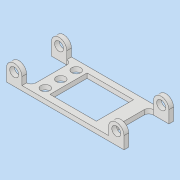
# Autodesk Inventor part: RelayHolder
Saved by Autodesk Inventor 2017 (Build 210142000, 142)
## iProperties
Created: 2018-03-03
Part Number: RelayHolder
Material: ABS Plastic
Document SubType Name: Modeling
Designer: Derek Wider
Density: 1.06 g/cm^3
Appearance: Smooth - White
Author: Derek Wider
Autodesk Inventor part; units mm, degrees
ref_plane "YZ Plane" through (0, 0, 0) normal (1, 0, 0) x (0, 1, 0)
ref_plane "XZ Plane" through (0, 0, 0) normal (0, 1, 0) x (-1, 0, 0)
ref_plane "XY Plane" through (0, 0, 0) normal (0, 0, 1) x (1, 0, 0)
sketch "Sketch1" plane through (0, 0, 0) normal (0, 1, 0) x (-1, 0, 0)
  line L0 (0, 0) -> (48.26, 0)
  line L1 (48.26, 0) -> (48.26, -20.32)
  line L2 (48.26, -20.32) -> (0, -20.32)
  line L3 (0, -20.32) -> (0, 0)
  line L4 (33.02, -2.6035) -> (13.97, -2.6035)
  line L5 (13.97, -2.6035) -> (13.97, -17.8435)
  line L6 (13.97, -17.8435) -> (33.02, -17.8435)
  line L7 (33.02, -17.8435) -> (33.02, -2.6035)
  dimension "d0" = 48.26
  dimension "d1" = 20.32
  dimension "d2" = 19.05
  dimension "d3" = 15.24
  dimension "d4" = 15.24
  dimension "d5" = 2.6035
  constraints: 16 end point, 4 parallel, 2 horizontal, 2 perpendicular
  measures "d0" distance of L1.end L2.end
  measures "d1" distance of L2.end L0.start
  measures "d2" distance of L4.start L4.end
  measures "d3" distance of L6.end L4.start
  measures "d4" distance between parallel lines of L1 L7
  measures "d5" distance between parallel lines of L0 L4
extrude "Extrusion1" add sketch "Sketch1" along normal blind 1.905
sketch "Sketch2" plane through (-48.26, 0, 0) normal (0, 0, 1) x (1, 0, 0)
  line L0 (48.26, 0) -> (0, 0) projected
  line L1 (48.26, 0) -> (48.26, 1.905) projected
  line L2 (0, 1.905) -> (48.26, 1.905) projected
  line L3 (0, 0) -> (0, 1.905) projected
  circle A0 centre (3.175, 5.08) radius 1.8415
  circle A1 centre (45.085, 5.08) radius 1.8415
  circle A2 centre (3.175, 5.08) radius 3.175
  circle A3 centre (45.085, 5.08) radius 3.175
  line L4 (0, 1.905) -> (48.26, 1.905) projected
  line L5 (0, 0) -> (0, 1.905) projected
  line L6 (0, 5.08) -> (0, 1.905)
  line L7 (6.35, 5.08) -> (6.35, 1.905)
  line L8 (48.26, 1.905) -> (0, 1.905) projected
  line L9 (48.26, 5.08) -> (48.26, 1.905)
  line L10 (41.91, 5.08) -> (41.91, 1.905)
  dimension "d8" = 3.683
  dimension "d9" = 41.91
  dimension "d10" = 6.35
  constraints: 8 end point, 5 tangent, 4 centre point, 4 point on circle, 2 coincident, 2 equal radius, 2 point on line, 1 horizontal alignment, 1 parallel, 1 perpendicular, 1 vertical
  measures "d8" diameter of A0
  measures "d9" distance of A1.centre A0.centre
  measures "d10" diameter of A2
extrude "Extrusion2" add sketch "Sketch2" against normal blind 1.905 contours L2 A3 L9 | L6 A2 L2 | L2 L10 A3 | A3 | A2 L7 L2 | A2
sketch "Sketch3" plane through (0, 0, -20.32) normal (0, 0, -1) x (-1, 0, 0)
  circle A0 centre (3.175, 5.08) radius 1.8415 projected
  arc A1 (6.35, 5.08) -> (0, 5.08) centre (3.175, 5.08) ccw projected
  line L0 (0, 5.08) -> (0, 1.905) projected
  line L1 (6.35, 1.905) -> (0, 1.905) projected
  line L2 (6.35, 1.905) -> (6.35, 5.08) projected
  circle A2 centre (45.085, 5.08) radius 1.8415 projected
  line L3 (48.26, 1.905) -> (41.91, 1.905) projected
  line L4 (48.26, 1.905) -> (48.26, 5.08) projected
  arc A3 (48.26, 5.08) -> (41.91, 5.08) centre (45.085, 5.08) ccw projected
  line L5 (41.91, 5.08) -> (41.91, 1.905) projected
  point P0 (0, 0)
extrude "Extrusion3" add sketch "Sketch3" against normal blind 1.905
sketch "Sketch4" plane through (0, 1.905, 0) normal (0, 1, 0) x (1, 0, 0)
  line L0 (-33.02, 2.6035) -> (-33.02, 17.8435) construction
  circle A0 centre (-36.195, 16.5735) radius 1.8415
  circle A1 centre (-36.195, 10.2235) radius 1.8415
  circle A2 centre (-36.195, 3.8735) radius 1.8415
  line L1 (-36.195, 16.5735) -> (-36.195, 10.2235) construction
  line L2 (-36.195, 10.2235) -> (-36.195, 3.8735) construction
  line L3 (-13.97, 2.6035) -> (-33.02, 2.6035) construction
  point P0 (0, 0)
  dimension "d18" = 3.683
  dimension "d19" = 3.175
  dimension "d20" = 6.35
  dimension "d21" = 1.27
  constraints: 4 end point, 3 centre point, 2 collinear, 2 equal radius, 2 vertical alignment, 1 vertical
  measures "d18" diameter of A2
  measures "d19" distance from line of L0 L2.end
  measures "d20" distance of L1.end L2.end
  measures "d21" distance from line of L3 L2.end
extrude "Extrusion4" cut sketch "Sketch4" against normal through all
sketch "Sketch5" plane through (0, 1.905, 0) normal (0, 1, 0) x (1, 0, 0)
  line L0 (-48.26, 18.415) -> (-41.91, 18.415) projected
  line L1 (-41.91, 1.905) -> (-48.26, 1.905) projected
  line L2 (0, 1.905) -> (-6.35, 1.905) projected
  line L3 (-6.35, 18.415) -> (0, 18.415) projected
  line L4 (-41.91, 18.415) -> (-48.26, 18.415) projected
  line L5 (-48.26, 18.415) -> (-40.005, 18.415)
  line L6 (-40.005, 18.415) -> (-40.005, 1.905)
  line L7 (-40.005, 1.905) -> (-48.26, 1.905)
  line L8 (-48.26, 1.905) -> (-48.26, 18.415)
  line L9 (0, 1.905) -> (-8.255, 1.905)
  line L10 (-8.255, 1.905) -> (-8.255, 18.415)
  line L11 (-8.255, 18.415) -> (0, 18.415)
  line L12 (0, 18.415) -> (0, 1.905)
  point P0 (0, 0)
  dimension "d24" = 8.255
  constraints: 16 end point, 4 parallel, 2 horizontal, 2 perpendicular, 2 point on line, 1 collinear
  measures "d24" distance of L0.start L5.end
extrude "Extrusion5" cut sketch "Sketch5" against normal through all
fillet "Fillet1" radius 1.905 4 edges at (-40.005, 0.9525, -18.415) (-40.005, 0.9525, -1.905) (-8.255, 0.9525, -1.905) (-8.255, 0.9525, -18.415)
body "Solid1"
